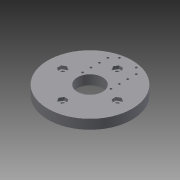
# Autodesk Inventor part: bowl_ax12_support_v2
Saved by Autodesk Inventor 2014 (Build 180170000, 170)
## iProperties
Created: 2014-01-13
Part Number: bowl_ax12_support_v2
Material: Générique
Document SubType Name: Modeling
Designer: helly
Density: 1 g/cm^3
Appearance: Par défaut
Author: helly
Autodesk Inventor part; units mm, degrees
ref_plane "YZ Plane" through (0, 0, 0) normal (1, 0, 0) x (0, 1, 0)
ref_plane "XZ Plane" through (0, 0, 0) normal (0, 1, 0) x (-1, 0, 0)
ref_plane "XY Plane" through (0, 0, 0) normal (0, 0, 1) x (1, 0, 0)
sketch "Esquisse1" plane through (0, 0, 0) normal (0, 0, 1) x (1, 0, 0)
  circle A0 centre (0, 0) radius 40
  circle A1 centre (0, 0) radius 12
  line L0 (0, 0) -> (-13.5, 0) construction
  line L1 (-13.5, 0) -> (-13.5, 6.5) construction
  line L2 (-13.5, 6.5) -> (-13.5, 14.5) construction
  line L3 (-13.5, 14.5) -> (-13.5, 22.5) construction
  line L4 (-13.5, 22.5) -> (-13.5, 30.5) construction
  line L5 (0, 0) -> (0, 36) construction
  line L6 (0, 36) -> (-8, 36) construction
  circle A2 centre (-13.5, 6.5) radius 1
  circle A3 centre (-13.5, 14.5) radius 1
  circle A4 centre (-13.5, 22.5) radius 1
  circle A5 centre (-13.5, 30.5) radius 1
  circle A6 centre (-8, 36) radius 1
  circle A7 centre (13.5, 6.5) radius 1
  circle A8 centre (13.5, 14.5) radius 1
  circle A9 centre (13.5, 22.5) radius 1
  circle A10 centre (13.5, 30.5) radius 1
  circle A11 centre (8, 36) radius 1
  line L7 (0, 0) -> (40, 0) construction
  line L8 (12, 0) -> (40, 0) construction
  circle A12 centre (26, 0) radius 2
  circle A13 centre (0, 26) radius 2
  circle A14 centre (-26, 0) radius 2
  circle A15 centre (0, -26) radius 2
  line L9 (0, 0) -> (0, -26) construction
  dimension "d0" = 80
  dimension "d1" = 24
  dimension "d2" = 13.5
  dimension "d3" = 6.5
  dimension "d4" = 8
  dimension "d5" = 8
  dimension "d6" = 8
  dimension "d7" = 36
  dimension "d8" = 8
  dimension "d9" = 2
  dimension "d25" = 4
  dimension "d28" = 360
  dimension "d39" = 26
  constraints: 20 end point, 14 centre point, 7 coincident, 5 symmetric about line, 4 collinear, 4 equal radius, 3 perpendicular, 2 horizontal alignment, 2 parallel, 1 horizontal, 1 midpoint, 1 point on line, 18 other
  measures "d2" distance of L0.start L0.end
  measures "d3" distance of L0.end L1.end
  measures "d4" distance of L1.end L2.end
  measures "d5" distance of L2.end L3.end
  measures "d6" distance of L3.end L4.end
  measures "d7" distance of L0.start L5.end
  measures "d8" distance of L5.end L6.end
  measures "d9" diameter of A2
  measures "d25" diameter of A12
  measures "d39" distance of L0.start L9.end
extrude "Extrusion3" add sketch "Esquisse1" along normal blind 9
sketch "Esquisse5" plane through (0, 0, 9) normal (0, 0, 1) x (1, 0, 0)
  circle A0 centre (0, 0) radius 12 projected
  circle A1 centre (0, -26) radius 2 projected
  circle A2 centre (-26, 0) radius 2 projected
  circle A3 centre (0, 26) radius 2 projected
  circle A4 centre (26, 0) radius 2 projected
  circle A5 centre (0, 0) radius 40 projected
  line L0 (0, 0) -> (40, 0) construction
  line L1 (29.5, 2.0207) -> (29.5, -2.0207)
  line L2 (29.5, -2.0207) -> (26, -4.0415)
  line L3 (26, -4.0415) -> (22.5, -2.0207)
  line L4 (22.5, -2.0207) -> (22.5, 2.0207)
  line L5 (22.5, 2.0207) -> (26, 4.0415)
  line L6 (26, 4.0415) -> (29.5, 2.0207)
  line L7 (22.5, 2.0207) -> (29.5, 2.0207) construction
  line L8 (-2.0207, 29.5) -> (2.0207, 29.5)
  line L9 (2.0207, 29.5) -> (4.0415, 26)
  line L10 (4.0415, 26) -> (2.0207, 22.5)
  line L11 (2.0207, 22.5) -> (-2.0207, 22.5)
  line L12 (-2.0207, 22.5) -> (-4.0415, 26)
  line L13 (-4.0415, 26) -> (-2.0207, 29.5)
  line L14 (-29.5, -2.0207) -> (-29.5, 2.0207)
  line L15 (-29.5, 2.0207) -> (-26, 4.0415)
  line L16 (-26, 4.0415) -> (-22.5, 2.0207)
  line L17 (-22.5, 2.0207) -> (-22.5, -2.0207)
  line L18 (-22.5, -2.0207) -> (-26, -4.0415)
  line L19 (-26, -4.0415) -> (-29.5, -2.0207)
  line L20 (2.0207, -29.5) -> (-2.0207, -29.5)
  line L21 (-2.0207, -29.5) -> (-4.0415, -26)
  line L22 (-4.0415, -26) -> (-2.0207, -22.5)
  line L23 (-2.0207, -22.5) -> (2.0207, -22.5)
  line L24 (2.0207, -22.5) -> (4.0415, -26)
  line L25 (4.0415, -26) -> (2.0207, -29.5)
  dimension "d50" = 7
  dimension "d53" = 360
  constraints: 52 end point, 2 perpendicular, 1 coincident, 1 horizontal, 1 horizontal alignment, 63 other
  measures "d50" distance of L4.end L1.start
extrude "Extrusion7" cut sketch "Esquisse5" against normal blind 3 contours L1 L2 L3 L4 L5 L6 | L8 L9 L10 L11 L12 L13 | L14 L15 L16 L17 L18 L19 | L20 L21 L22 L23 L24 L25
